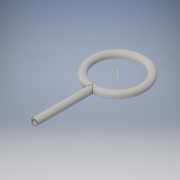
# Autodesk Inventor part: catapultLoop
Saved by Autodesk Inventor 2016 SP1 (Build 200210100, 210)
## iProperties
Created: 2016-01-16
Part Number: catapultLoop
Material: Generic
Document SubType Name: Modeling
Designer: steele
Density: 1 g/cm^3
Appearance: Default
Author: steele
Autodesk Inventor part; units mm, degrees
ref_plane "XZ Plane" through (0, 0, 0) normal (0, 1, 0) x (-1, 0, 0)
sketch "Sketch3" plane through (0, 0, 0) normal (1, 0, 0) x (0, 1, 0)
  circle A0 centre (0, -101.6) radius 13.97
  line L0 (-19.558, 0) -> (19.558, 0) projected
  circle A1 centre (0, -101.6) radius 9.525
  point P0 (0, 0)
  dimension "d6" = 27.94
  dimension "d7" = 101.6
  dimension "d13" = 19.05
  constraints: 2 centre point, 1 coincident
  measures "d6" diameter of A0
  measures "d7" distance of point (0, 0) A0.centre
  measures "d13" diameter of A1
revolve "Revolution3" add sketch "Sketch3" angle 360 about axis through (0, -10, 0) along (0, 1, 0)
ref_plane "Work Plane3" through (0, 0, 101.6) normal (0, 0, 1) x (1, 0, 0)
sketch "Sketch5" plane through (0, 0, 101.6) normal (0, 0, 1) x (1, 0, 0)
  circle A0 centre (0, 0) radius 13.97
  circle A1 centre (0, 0) radius 9.525
  dimension "d17" = 27.94
  dimension "d18" = 19.05
  constraints: 2 centre point, 2 coincident
  measures "d17" diameter of A0
  measures "d18" diameter of A1
extrude "Extrusion2" add sketch "Sketch5" along normal blind 240.03
ref_plane "Work Plane4" through (13.97, 0, 101.6) normal (1, 0, 0) x (0, 1, 0)
sketch "Sketch6" plane through (13.97, 0, 101.6) normal (1, 0, 0) x (0, 1, 0)
  circle A0 centre (0, 214.63) radius 3.302
  line L0 (13.97, 240.03) -> (-13.97, 240.03) projected
  point P0 (0, -101.6)
  dimension "d21" = 6.604
  dimension "d22" = 25.4
  constraints: 1 centre point
  measures "d21" diameter of A0
  measures "d22" distance from line of A0.centre L0
extrude "Extrusion3" cut sketch "Sketch6" against normal through all
equation "\"d6\" = ballHolderPipeOutsideDiam"
equation "\"d7\" = ballHolderLoopRadius"
equation "\"d13\" = ballHolderPipeInsideDiam"
equation "\"d17\" = ballHolderPipeOutsideDiam"
equation "\"d18\" = ballHolderPipeInsideDiam"
equation "\"d19\" = ballHolderLoopHandleLength"
equation "\"d21\" = ballHolderAxelDiam"
equation "\"d22\" = ballHolderAxelDistanceFromEnd"
equation "\"d23\" = ballHolderLoopHandleLength"
equation "\"ballHolderLoopDiam\" = 203.2"
equation "\"xxx\" = 0.5 * ballHolderLoopDiam + ballHolderLoopHandleLength"
equation "\"ballHolderPipeInsideDiam\" = 19.05"
equation "\"ballHolderPipeOutsideDiam\" = 27.94"
equation "\"ballHolderLoopRadius\" = 0.5 * ballHolderLoopDiam"
equation "\"d16\" = ballHolderLoopRadius"
equation "\"ballHolderAxelDiam\" = 6.604"
equation "\"ballHolderAxelDistanceFromEnd\" = 25.4"
equation "\"ballHolderLoopHandleLength\" = 240.03"
body "Solid2"
